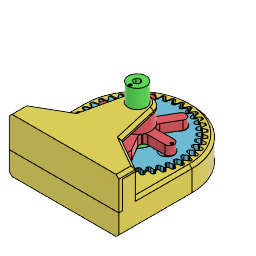
Dual ACG gear train - Trapezoidal Tooth  A2 (Autodesk Fusion 360 design; units mm, degrees)
Autodesk Fusion 360 part; units mm, degrees
note: some values were not read from the file. Set by a fixed rule: which face or edge a step refers to.
(part 1 of 4)
sketch "Disc-D108-E1_215-Dp4-N40-Phase2-20260428-091808-Disc2" plane through (0, 0, 0) normal (0, 0, 1) x (1, 0, 0) in component "DXF profiles - MEVirtuoso"